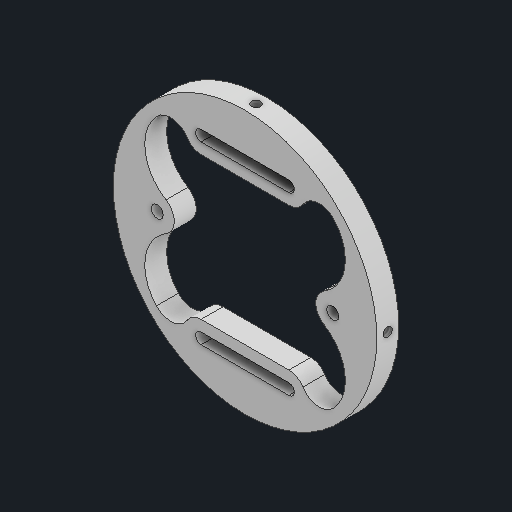
# Autodesk Inventor part: DeploymentBulkhead
Saved by Autodesk Inventor 2026.2 (Build 302298010, 298A)
## iProperties
Created: 2026-03-08
Part Number: DeploymentBulkhead
Material: Generic
Document SubType Name: Modeling
Designer: grhfa
Density: 1 g/cm^3
Appearance: Default
Author: grhfa
Autodesk Inventor part; units mm, degrees
ref_plane "YZ Plane" through (0, 0, 0) normal (1, 0, 0) x (0, 1, 0)
ref_plane "XY Plane" through (0, 0, 0) normal (0, 0, 1) x (1, 0, 0)
sketch "Sketch1" plane through (0, 0, 0) normal (0, 0, 1) x (1, 0, 0)
  circle A0 centre (0, 0) radius 38.1
  line L0 (-12.7, 25.4) -> (12.7, 25.4) construction
  line L1 (-12.7, 23.8125) -> (12.7, 23.8125)
  line L2 (12.7, 26.9875) -> (-12.7, 26.9875)
  arc A1 (-12.7, 26.9875) -> (-12.7, 23.8125) centre (-12.7, 25.4) ccw
  arc A2 (12.7, 23.8125) -> (12.7, 26.9875) centre (12.7, 25.4) ccw
  line L3 (0, 38.1) -> (0, -38.1) construction
  line L4 (-38.1, 0) -> (38.1, 0) construction
  line L5 (-12.7, -25.4) -> (12.7, -25.4) construction
  line L6 (-12.7, -23.8125) -> (12.7, -23.8125)
  line L7 (12.7, -26.9875) -> (-12.7, -26.9875)
  arc A3 (-12.7, -23.8125) -> (-12.7, -26.9875) centre (-12.7, -25.4) ccw
  arc A4 (12.7, -26.9875) -> (12.7, -23.8125) centre (12.7, -25.4) ccw
  point P0 (0, 25.4)
  point P1 (0, -25.4)
  dimension "d0" = 76.2
  dimension "d1" = 25.4
  dimension "d2" = 1.5875
  dimension "d3" = 25.4
  constraints: 20 end point, 12 point on circle, 7 symmetric about line, 5 centre point, 4 midpoint, 4 tangent, 1 coincident, 1 horizontal, 1 parallel, 1 perpendicular, 1 point on line, 1 vertical, 2 other
  measures "d0" diameter of A0
  measures "d1" distance between parallel lines of L4 L0
  measures "d2" radius of A2
  measures "d3" distance of L2.start L2.end
extrude "Extrusion1" add sketch "Sketch1" along normal mid plane 6.35
sketch "Sketch2" plane through (0, 0, 3.175) normal (0, 0, 1) x (1, 0, 0)
  circle A0 centre (0, 0) radius 38.1 construction
  line L0 (0, 38.1) -> (0, -38.1) construction
  point P0 (-25.4, 0)
  point P1 (25.4, 0)
  dimension "d8" = 25.4
  constraints: 2 end point, 2 midpoint, 2 point on circle, 1 horizontal alignment, 1 symmetric about line, 1 vertical
  measures "d8" distance from line of L0 point (-25.4, 0)
hole "Hole1" at (-25.4, 0, 3.175) at (25.4, 0, 3.175) direction (0, 0, -1) diameter 3.5052 end through all
sketch "Sketch3" plane through (0, 0, 3.175) normal (0, 0, 1) x (1, 0, 0)
  circle A0 centre (25.4, 0) radius 1.7526 construction
  circle A1 centre (-25.4, 0) radius 1.7526 construction
  circle A2 centre (0, 0) radius 38.1 construction
  line L0 (12.7, -26.9875) -> (-12.7, -26.9875) construction
  arc A3 (-12.7, -23.8125) -> (-12.7, -26.9875) centre (-12.7, -25.4) ccw construction
  line L1 (-12.7, -23.8125) -> (12.7, -23.8125) construction
  arc A4 (12.7, -26.9875) -> (12.7, -23.8125) centre (12.7, -25.4) ccw construction
  arc A5 (-12.7, 26.9875) -> (-12.7, 23.8125) centre (-12.7, 25.4) ccw construction
  line L2 (-12.7, 26.9875) -> (12.7, 26.9875) construction
  arc A6 (12.7, 23.8125) -> (12.7, 26.9875) centre (12.7, 25.4) ccw construction
  line L3 (12.7, 23.8125) -> (-12.7, 23.8125) construction
  line L4 (12.7, 30.1625) -> (-12.7, 30.1625)
  arc A7 (-12.7, 30.1625) -> (-12.7, 20.6375) centre (-12.7, 25.4) ccw
  line L5 (-12.7, 20.6375) -> (12.7, 20.6375)
  arc A8 (12.7, 20.6375) -> (12.7, 30.1625) centre (12.7, 25.4) ccw
  circle A9 centre (-25.4, 0) radius 4.9276
  circle A10 centre (25.4, 0) radius 4.9276
  line L6 (12.7, -20.6375) -> (-12.7, -20.6375)
  arc A11 (-12.7, -20.6375) -> (-12.7, -30.1625) centre (-12.7, -25.4) ccw
  line L7 (-12.7, -30.1625) -> (12.7, -30.1625)
  arc A12 (12.7, -30.1625) -> (12.7, -20.6375) centre (12.7, -25.4) ccw
  circle A13 centre (0, 0) radius 34.925
  arc A14 (-25.6248, 23.7303) -> (-22.8581, 4.2213) centre (-16.3067, 15.1011) ccw
  arc A15 (-22.8581, -4.2213) -> (-25.6248, -23.7303) centre (-16.3067, -15.1011) ccw
  arc A16 (22.8581, 4.2213) -> (25.6248, 23.7303) centre (16.3067, 15.1011) ccw
  arc A17 (25.6248, -23.7303) -> (22.8581, -4.2213) centre (16.3067, -15.1011) ccw
  arc A18 (-25.6248, -23.7303) -> (-16.7431, -22.8831) centre (-21.5072, -19.9172) ccw
  arc A19 (16.7431, -22.8831) -> (25.6248, -23.7303) centre (21.5072, -19.9172) ccw
  arc A20 (-16.7431, 22.8831) -> (-25.6248, 23.7303) centre (-21.5072, 19.9172) ccw
  arc A21 (25.6248, 23.7303) -> (16.7431, 22.8831) centre (21.5072, 19.9172) ccw
  dimension "d16" = 3.175
  dimension "d17" = 3.175
  dimension "d18" = 3.175
  dimension "d19" = 3.175
  dimension "d20" = 3.175
  dimension "d21" = 12.7
  constraints: 36 point on circle, 16 tangent, 15 centre point, 8 end point, 2 horizontal alignment, 2 vertical alignment, 6 other
  measures "d16" distance between parallel lines of L2 L4
  measures "d17" radial gap between concentric circles of A1 A9
  measures "d18" radial gap between concentric circles of A0 A10
  measures "d19" distance between parallel lines of L1 L6
  measures "d20" radial gap between concentric circles of A2 A13
  measures "d21" radius of A16
extrude "Extrusion2" cut sketch "Sketch3" against normal through all contours A21 A16 A10 A17 A19 A12 L6 A11 A18 A15 A9 A14 A20 A7 L5 A8
ref_plane "Work Plane1" through (0, 38.1, 0) normal (0, 1, 0) x (-1, 0, 0)
sketch "Sketch4" plane through (0, 38.1, 0) normal (0, 1, 0) x (-1, 0, 0)
  point P0 (0, 0)
  point P1 (0, 0)
  constraints: 1 coincident
hole "Hole2" at (0, 38.1, 0) direction (0, -1, 0) diameter 2.6416 depth 6.35 tip angle 118 thread size "6-32 UNC" class "2B" standard "ANSI Unified Screw Threads"
pattern_circular "Circular Pattern1" count 4 over 360 about axis through (0, 0, 0) along (0, 0, 1) of "Hole2"
body "Solid1"
